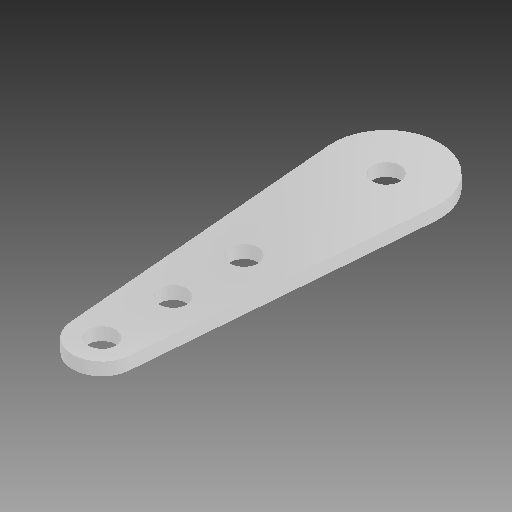
# Autodesk Inventor part: Master
Saved by Autodesk Inventor 2023 (Build 270158000, 158)
## iProperties
Created: 2020-11-18
Part Number: Master
Material: Aluminum 6061
Document SubType Name: Modeling
Density: 2.7 g/cm^3
Appearance: Aluminum - Dark
Mass: 5.32372 g
Surface Area: 22.0741 cm^2
Volume: 1.97175 cm^3
Sheet Metal Rule: Default
Mass: 8.32687 g
Surface Area: 34.778 cm^2
Volume: 3.08403 cm^3
Revision Number: 0
Document SubType Name: Sheet Metal
Autodesk Inventor part; units mm, degrees
ref_plane "YZ Plane" through (0, 0, 0) normal (1, 0, 0) x (0, 1, 0)
ref_plane "XZ Plane" through (0, 0, 0) normal (0, 1, 0) x (-1, 0, 0)
ref_plane "XY Plane" through (0, 0, 0) normal (0, 0, 1) x (1, 0, 0)
sketch "Sketch1" plane through (0, 0, 0) normal (0, 1, 0) x (-1, 0, 0)
  line L0 (25.4, 0) -> (-25.4, 0) construction
  circle A0 centre (25.4, 0) radius 2.4892
  line L1 (0, 0) -> (0, 50.8) construction
  circle A1 centre (0, 25.4) radius 2.4892
  circle A2 centre (0, 38.1) radius 2.4892
  circle A3 centre (0, 50.8) radius 2.4892
  circle A4 centre (0, 0) radius 9.525
  circle A5 centre (0, 50.8) radius 5.2705
  circle A6 centre (-25.4, 0) radius 5.2705
  circle A7 centre (25.4, 0) radius 5.2705
  line L2 (26.2828, -5.196) -> (1.5954, -9.3904)
  line L3 (-1.5954, -9.3904) -> (-26.2828, -5.196)
  line L4 (26.2828, 5.196) -> (16.1511, 6.9174)
  line L5 (-26.2828, 5.196) -> (-16.1511, 6.9174)
  line L6 (9.4915, 0.7977) -> (5.252, 51.2414)
  line L7 (-9.4915, 0.7977) -> (-5.252, 51.2414)
  arc A8 (8.255, 15.5101) -> (16.1511, 6.9174) centre (17.7466, 16.3078) ccw
  arc A9 (-16.1511, 6.9174) -> (-8.255, 15.5101) centre (-17.7466, 16.3078) ccw
  circle A10 centre (12.7, 0) radius 2.4892
  circle A11 centre (0, 0) radius 2.4892
  circle A12 centre (-12.7, 0) radius 2.4892
  circle A13 centre (-25.4, 0) radius 2.4892
  line L8 (-9.4915, -0.7977) -> (-5.252, -51.2414)
  line L9 (9.4915, -0.7977) -> (5.252, -51.2414)
  arc A14 (-5.252, -51.2414) -> (5.252, -51.2414) centre (0, -50.8) ccw
  circle A15 centre (0, -50.8) radius 2.4892
  circle A16 centre (0, -38.1) radius 2.4892
  circle A17 centre (0, -25.4) radius 2.4892
  arc A18 (16.1511, -6.9174) -> (8.255, -15.5101) centre (17.7466, -16.3078) ccw
  arc A19 (-8.255, -15.5101) -> (-16.1511, -6.9174) centre (-17.7466, -16.3078) ccw
  circle A20 centre (-25.4, 0) radius 2.4892
  point P0 (8.9772, -6.9173)
  point P1 (-8.9772, -6.9173)
  dimension "d1" = 4.9784
  dimension "d11" = 25.4
  dimension "d18" = 12.7
  dimension "d28" = 19.05
  dimension "d29" = 10.541
  dimension "d30" = 9.525
  dimension "d33" = 12.7
  dimension "d38" = 25.4
  dimension "d47" = 12.7
  dimension "d52" = 25.4
  constraints: 24 tangent, 22 point on circle, 21 centre point, 20 end point, 9 coincident, 9 equal radius, 8 point on line, 3 vertical, 2 horizontal, 2 horizontal alignment, 2 vertical alignment, 1 equal length, 1 midpoint, 17 other
  measures "d1" diameter of A0
  measures "d11" distance of point (0, 0) A1.centre
  measures "d18" distance of A1.centre A2.centre
  measures "d28" diameter of A4
  measures "d29" diameter of A5
  measures "d30" radius of A8
  measures "d33" distance of A0.centre A10.centre
  measures "d38" distance of point (0, 0) A0.centre
  measures "d47" distance of A15.centre A16.centre
  measures "d52" distance of A11.centre A17.centre
extrude "Full Gusset" add sketch "Sketch1" along normal blind 2.286
extrude "Minus Top" cut sketch "Sketch1" along normal blind 2.286 contours L2 L9 A14 L8 L3 A4 | L2 A18 L9 | L8 A19 L3
extrude "Minus Left" cut sketch "Sketch1" along normal blind 2.286 contours A4 L6 A8 L4 A7 L2 L9 | L9 L2 A4 | A7
mirror "Mirror1" about plane through (0, 0, 0) normal (1, 0, 0) of "Minus Left"
sketch "Sketch3" plane through (0, 2.286, 0) normal (0, 1, 0) x (1, 0, 0)
  circle A0 centre (0, 0) radius 2.4892 projected
  point P0 (0, 0)
extrude "Extrusion5" [suppressed]
equation "\"BendRadius\" = Thickness"
equation "\"BendReliefWidth\" = Thickness"
equation "\"BendReliefDepth\" = 0.5 * Thickness"
equation "\"CornerReliefSize\" = 4 * Thickness"
equation "\"MinimumRemnant\" = 2 * Thickness"
equation "\"TransitionRadius\" = BendRadius"
equation "\"JacobiRadiusSize\" = BendRadius"
equation "\"GapSize\" = Thickness"
equation "\"Thickness\" = 2.286"
body "Solid2"
